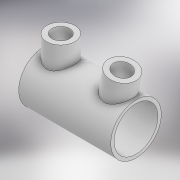
# Autodesk Inventor part: JuntaRodilla
Saved by Autodesk Inventor 2021 (Build 250183000, 183)
## iProperties
Created: 2024-02-19
Part Number: JuntaRodilla
Material: Generic
Document SubType Name: Modeling
Designer: Martin
Density: 1 g/cm^3
Appearance: Default
Author: Martin
Autodesk Inventor part; units mm, degrees
ref_plane "YZ Plane" through (0, 0, 0) normal (1, 0, 0) x (0, 1, 0)
ref_plane "XZ Plane" through (0, 0, 0) normal (0, 1, 0) x (-1, 0, 0)
ref_plane "XY Plane" through (0, 0, 0) normal (0, 0, 1) x (1, 0, 0)
sketch "Sketch1" plane through (0, 0, 0) normal (1, 0, 0) x (0, 1, 0)
  circle A0 centre (0, 0) radius 19.5
  circle A1 centre (0, 0) radius 22.5
  dimension "d0" = 39
  dimension "d1" = 45
  constraints: 2 centre point, 2 coincident
  measures "d0" diameter of A0
  measures "d1" diameter of A1
extrude "Extrusion1" add sketch "Sketch1" along normal mid plane 82
ref_plane "Work Plane1" through (0, 40, 0) normal (0, 1, 0) x (-1, 0, 0)
sketch "Sketch2" plane through (0, 40, 0) normal (0, 1, 0) x (-1, 0, 0)
  circle A0 centre (26, 0) radius 12.5
  circle A1 centre (26, 0) radius 7.9
  line L0 (41, -22.5) -> (41, 22.5) projected
  point P0 (0, 0)
  dimension "d6" = 25
  dimension "d7" = 15.8
  dimension "d19" = 15
  constraints: 2 centre point, 1 coincident
  measures "d6" diameter of A0
  measures "d7" diameter of A1
  measures "d19" distance from line of L0 A0.centre
extrude "Extrusion2" add sketch "Sketch2" against normal up to surface round surface about axis through (0, 0, 0) along (1, 0, 0) radius 22.5 far side no
sketch "Sketch3" plane through (0, 40, 0) normal (0, 1, 0) x (-1, 0, 0)
  line L0 (41, 22.5) -> (-41, 22.5) projected
  line L1 (-25, 22.5) -> (-25, -21.8926)
  line L2 (41, 22.5) -> (-41, 22.5) projected
  point P0 (0, 0)
  dimension "d16" = 25
  constraints: 2 end point, 1 perpendicular, 1 point on line
  measures "d16" distance from line of L1 point (0, 0)
ref_plane "Work Plane3" through (25, 40, 22.5) normal (0.1736482, 0.9848078, 0) x (0, 0, -1)
sketch "Sketch4" plane through (25, 40, 22.5) normal (0.1736482, 0.9848078, 0) x (0, 0, -1)
  ellipse E0 centre (22.5, 50.2252) end of major axis (14.6, 50.2252) minor radius 7.78 projected
  circle A0 centre (22.5, -3.7748) radius 7.9
  circle A1 centre (22.5, -3.7748) radius 12.5
  ellipse E1 centre (22.5, 50.2252) end of major axis (10, 50.2252) minor radius 12.3101 projected
  point P0 (22.5, 17.6743)
  dimension "d11" = 54
  dimension "d12" = 15.8
  dimension "d13" = 25
  constraints: 3 coincident, 2 centre point, 2 other
  measures "d11" distance of point (22.5, -3.775) point (22.5, 50.225)
  measures "d12" diameter of A0
  measures "d13" diameter of A1
extrude "Extrusion3" add sketch "Sketch4" against normal up to surface contours A1 round surface about axis through (0, 0, 0) along (1, 0, 0) radius 22.5 far side no
body "Solid1"
